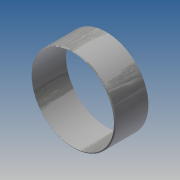
# Autodesk Inventor part: A1-19027-100-02 36in pipe
Saved by Autodesk Inventor 2017.3 (Build 213257000, 257)
## iProperties
Created: 2019-10-16
Part Number: A1-19027-100-02 36in pipe
Material: Steel, Mild
Description: 36" XS x 14 17/32" PIPE, X65M
Document SubType Name: Modeling
Designer: GVD
Density: 7.85 g/cm^3
Appearance: Steel
Mass: 102102 g
Surface Area: 21301.9 cm^2
Volume: 13006.6 cm^3
Author: GVD
Autodesk Inventor part; units mm, degrees
ref_plane "YZ Plane" through (0, 0, 0) normal (1, 0, 0) x (0, 1, 0)
ref_plane "XZ Plane" through (0, 0, 0) normal (0, 1, 0) x (-1, 0, 0)
ref_plane "XY Plane" through (0, 0, 0) normal (0, 0, 1) x (1, 0, 0)
sketch "Sketch1" plane through (0, 0, 0) normal (0, 0, 1) x (1, 0, 0)
  circle A0 centre (0, 0) radius 457.2
  circle A1 centre (0, 0) radius 444.5
  dimension "d0" = 914.4
  dimension "d1" = 889
  constraints: 2 centre point, 2 coincident
  measures "d0" diameter of A0
  measures "d1" diameter of A1
extrude "Extrusion1" add sketch "Sketch1" along normal blind 369.0375
chamfer "Chamfer1" distance 11.1125 angle 37.5 1 edges at (-457.2, 0, 0) measured on face at (-456.7, 0, 0)
chamfer "Chamfer2" distance 11.1125 angle 37.5 1 edges at (-457.2, 0, 369.0375) measured on face at (-456.7, 0, 369.0375)
equation "\"d7\" = d4"
equation "\"d9\" = d6"
equation "\"d4\" = 11.1125"
equation "\"d6\" = 37.5deg"
body "Solid1"
